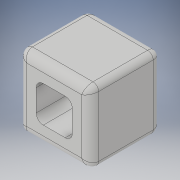
# Autodesk Inventor part: Square-Circle-Adapter V2D1
Saved by Autodesk Inventor 2017 (Build 210142000, 142)
## iProperties
Created: 2018-01-23
Part Number: Square-Circle-Adapter V2D1
Material: Generic
Document SubType Name: Modeling
Designer: Tripl_000
Density: 1 g/cm^3
Appearance: Default
Author: Tripl_000
Autodesk Inventor part; units mm, degrees
ref_plane "YZ Plane" through (0, 0, 0) normal (1, 0, 0) x (0, 1, 0)
ref_plane "XZ Plane" through (0, 0, 0) normal (0, 1, 0) x (-1, 0, 0)
ref_plane "XY Plane" through (0, 0, 0) normal (0, 0, 1) x (1, 0, 0)
sketch "Sketch1" plane through (0, 0, 0) normal (0, 0, 1) x (1, 0, 0)
  line L0 (-12.75, 12.75) -> (12.75, 12.75)
  line L1 (12.75, 12.75) -> (12.75, -12.75)
  line L2 (12.75, -12.75) -> (-12.75, -12.75)
  line L3 (-12.75, -12.75) -> (-12.75, 12.75)
  line L4 (-12.75, 12.75) -> (12.75, -12.75) construction
  line L5 (12.75, 12.75) -> (-12.75, -12.75) construction
  point P0 (0, 0)
  dimension "d0" = 25.5
  dimension "d1" = 25.5
  constraints: 12 end point, 2 midpoint, 2 parallel, 1 horizontal, 1 perpendicular
  measures "d0" distance of L0.start L0.end
  measures "d1" distance between parallel lines of L2 L0
extrude "Extrusion1" add sketch "Sketch1" along normal blind 25.4
sketch "Sketch2" plane through (0, 0, 25.4) normal (0, 0, 1) x (1, 0, 0)
  circle A0 centre (0, 0) radius 3
  dimension "d4" = 6
  constraints: 1 centre point, 1 coincident
  measures "d4" diameter of A0
extrude "Extrusion2" cut sketch "Sketch2" against normal through all
sketch "Sketch3" plane through (0, 0, 25.4) normal (0, 0, 1) x (1, 0, 0)
  line L0 (-6.4, 6.4) -> (6.4, 6.4)
  line L1 (6.4, 6.4) -> (6.4, -6.4)
  line L2 (6.4, -6.4) -> (-6.4, -6.4)
  line L3 (-6.4, -6.4) -> (-6.4, 6.4)
  line L4 (-6.4, 6.4) -> (6.4, -6.4) construction
  line L5 (6.4, 6.4) -> (-6.4, -6.4) construction
  point P0 (0, 0)
  dimension "d7" = 12.8
  dimension "d8" = 12.8
  constraints: 12 end point, 2 midpoint, 2 parallel, 1 horizontal, 1 perpendicular
  measures "d7" distance of L0.end L1.end
  measures "d8" distance of L0.start L0.end
extrude "Extrusion3" cut sketch "Sketch3" against normal blind 12.7
fillet "Fillet1" radius 2.5 4 edges at (6.4, 6.4, 19.05) (-6.4, 6.4, 19.05) (-6.4, -6.4, 19.05) (6.4, -6.4, 19.05)
fillet "Fillet2" radius 2 4 edges at (-12.75, 12.75, 12.7) (12.75, 12.75, 12.7) (-12.75, -12.75, 12.7) (12.75, -12.75, 12.7)
fillet "Fillet4" radius 3 8 edges at (12.1642, 12.1642, 0) (12.75, 0, 0) (12.1642, -12.1642, 0) (0, -12.75, 0) (-12.1642, -12.1642, 0) (-12.75, 0, 0) (-12.1642, 12.1642, 0) (0, 12.75, 0)
fillet "Fillet5" radius 3 8 edges at (12.1642, 12.1642, 25.4) (0, 12.75, 25.4) (-12.1642, 12.1642, 25.4) (-12.75, 0, 25.4) (-12.1642, -12.1642, 25.4) (0, -12.75, 25.4) (12.1642, -12.1642, 25.4) (12.75, 0, 25.4)
fillet "Fillet6" radius 6 1 edges at (-3, 0, 12.7)
body "Solid1"
